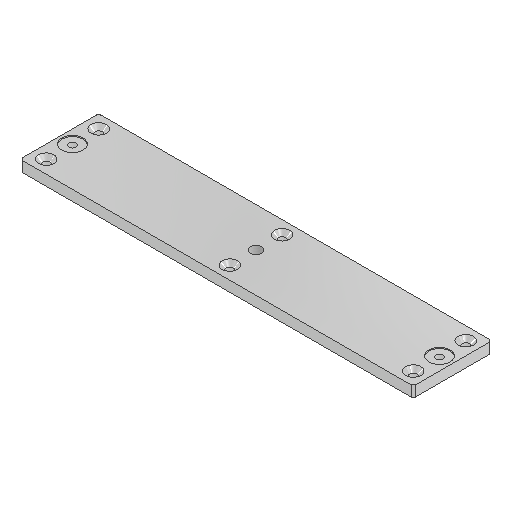
# Autodesk Inventor part: DLT-01-235B
Saved by Autodesk Inventor 2025.2 (Build 292293000, 293)
## iProperties
Company: Delta
Created: 2024-11-01
Part Number: DLT-01-235B
Material: Aluminio 1060
Document SubType Name: Modeling
Designer: Willian Pinheiro
Density: 2.7 g/cm^3
Appearance: Aluminum - Polished
Project: DLT
Description: Suporte Base Pressor B
Mass: 742.966 g
Surface Area: 663.177 cm^2
Volume: 275.172 cm^3
Acabamento: N/A
Dimensões: 10 x 75 x 375
Total: 1
Author: Willian Pinheiro
Revision Number: 00
Autodesk Inventor part; units mm, degrees
ref_plane "YZ Plane" through (0, 0, 0) normal (1, 0, 0) x (0, 1, 0)
ref_plane "XZ Plane" through (0, 0, 0) normal (0, 1, 0) x (-1, 0, 0)
ref_plane "XY Plane" through (0, 0, 0) normal (0, 0, 1) x (1, 0, 0)
sketch "Sketch1" plane through (0, 0, 0) normal (0, 0, 1) x (1, 0, 0)
  line L0 (-262.5, 0) -> (262.5, 0) construction
  line L1 (0, -52.5) -> (0, 52.5) construction
  line L2 (-187.5, 37.5) -> (187.5, 37.5)
  line L3 (187.5, 37.5) -> (187.5, -37.5)
  line L4 (187.5, -37.5) -> (-187.5, -37.5)
  line L5 (-187.5, -37.5) -> (-187.5, 37.5)
  point P0 (-175, 25)
  point P1 (175, 25)
  point P2 (-175, -25)
  point P3 (175, -25)
  point P4 (0, 0)
  point P5 (-175, 0)
  point P6 (175, 0)
  point P7 (0, 25)
  point P8 (0, -25)
  dimension "d0" = 375
  dimension "d1" = 75
  dimension "d3" = 350
  dimension "d30" = 12.5
  dimension "d45" = 12.5
  constraints: 8 end point, 4 symmetric about line, 3 point on line, 2 horizontal alignment, 2 midpoint, 2 parallel, 1 horizontal, 1 perpendicular, 1 vertical alignment, 2 other
  measures "d0" distance between parallel lines of L3 L5
  measures "d1" distance between parallel lines of L4 L2
  measures "d3" distance of point (175, 25) point (-175, 25)
  measures "d30" distance from line of L5 point (-175, 25)
  measures "d45" distance from line of L2 point (-175, 25)
extrude "Extrusion1" add sketch "Sketch1" against normal blind 10
hole "Hole1" at (-175, 25, 0) at (175, 25, 0) at (-175, -25, 0) at (175, -25, 0) at (0, 25, 0) at (0, -25, 0) direction (0, 0, -1) diameter 6.6 end through all countersink diameter 14.5 countersink angle 90 clearance for "Countersunk Flat Head Hex Socket Screw ISO 10642" size "M6" standard "ISO"
hole "Hole2" at (0, 0, 0) direction (0, 0, -1) diameter 10.647 end through all thread size "M12x1.25" class "6H" standard "ISO Metric profile"
hole "Hole3" at (-175, 0, 0) at (175, 0, 0) direction (0, 0, -1) diameter 20 depth 1
sketch "Sketch2" plane through (0, 0, -10) normal (0, 0, -1) x (-1, 0, 0)
  circle A0 centre (175, 0) radius 10 projected
  circle A1 centre (-175, 0) radius 10 projected
  point P0 (0, 0)
  constraints: 2 coincident
hole "Hole4" at (-175, 0, -10) at (175, 0, -10) direction (0, 0, 1) diameter 6.6 end through all countersink diameter 14.5 countersink angle 90 clearance for "Countersunk Flat Head Hex Socket Screw ISO 10642" size "M6" standard "ISO"
chamfer "Chamfer1" distance 2 angle 45 4 edges at (-187.5, 37.5, -5) (-187.5, -37.5, -5) (187.5, 37.5, -5) (187.5, -37.5, -5)
equation "\"d45\" = d30"
body "Solid1"
